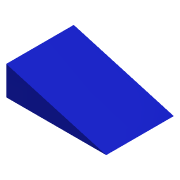
# Autodesk Inventor part: Wedge version 2
Saved by Autodesk Inventor 2015 (Build 190159000, 159)
## iProperties
Created: 2015-01-20
Part Number: Wedge version 2
Material: Generic
Document SubType Name: Modeling
Designer: Peter
Density: 1 g/cm^3
Appearance: Blue - Wall Paint - Glossy
Author: Peter
Autodesk Inventor part; units mm, degrees
ref_plane "YZ Plane" through (0, 0, 0) normal (1, 0, 0) x (0, 1, 0)
ref_plane "XZ Plane" through (0, 0, 0) normal (0, 1, 0) x (-1, 0, 0)
ref_plane "XY Plane" through (0, 0, 0) normal (0, 0, 1) x (1, 0, 0)
sketch "Sketch1" plane through (0, 0, 0) normal (0, 0, 1) x (1, 0, 0)
  line L0 (0, 0) -> (0, 38.1)
  line L1 (0, 38.1) -> (131.6736, 0)
  line L2 (131.6736, 0) -> (0, 0)
  dimension "d0" = 38.1
  dimension "d1" = 131.6736
  constraints: 6 end point, 1 perpendicular, 1 vertical
  measures "d0" distance of L0.start L0.end
  measures "d1" distance of L1.end L0.start
extrude "Extrusion1" add sketch "Sketch1" along normal blind 88.9
body "Solid1"
